Autodesk Inventor part; units mm, degrees
(part 3 of 3)
  circle A63 centre (27.5, -71.0469) radius 1.6 construction
  circle A64 centre (72.5, 11.9531) radius 1.6 construction
  circle A65 centre (27.5, 11.9531) radius 1.6 construction
  circle A66 centre (50, 69.0653) radius 1.6 construction
  arc A67 (58, 66.0653) -> (55, 66.0653) centre (56.5, 66.0653) ccw construction
  line L1375 (58, 66.0653) -> (58, 63.0653) construction
  arc A68 (55, 63.0653) -> (58, 63.0653) centre (56.5, 63.0653) ccw construction
  line L1376 (55, 63.0653) -> (45, 63.0653) construction
  arc A69 (42, 63.0653) -> (45, 63.0653) centre (43.5, 63.0653) ccw construction
  line L1377 (42, 63.0653) -> (42, 66.0653) construction
  arc A70 (45, 66.0653) -> (42, 66.0653) centre (43.5, 66.0653) ccw construction
  line L1378 (45, 66.0653) -> (55, 66.0653) construction
  circle A71 centre (50, 53.0653) radius 1.6 construction
  arc A72 (58, 50.0653) -> (55, 50.0653) centre (56.5, 50.0653) ccw construction
  line L1379 (58, 50.0653) -> (58, 47.0653) construction
  arc A73 (55, 47.0653) -> (58, 47.0653) centre (56.5, 47.0653) ccw construction
  line L1380 (55, 47.0653) -> (45, 47.0653) construction
  arc A74 (42, 47.0653) -> (45, 47.0653) centre (43.5, 47.0653) ccw construction
  line L1381 (42, 47.0653) -> (42, 50.0653) construction
  arc A75 (45, 50.0653) -> (42, 50.0653) centre (43.5, 50.0653) ccw construction
  line L1382 (45, 50.0653) -> (55, 50.0653) construction
  circle A76 centre (50, 24.7653) radius 5 construction
  circle A77 centre (50, -37.0469) radius 9.5 construction
  circle A78 centre (10, 22.9531) radius 1.6 construction
  circle A79 centre (10, -97.0469) radius 1.6 construction
  circle A80 centre (10, -97.0469) radius 1.6
  circle A81 centre (10, 47.9531) radius 1.6
  circle A82 centre (10, 22.9531) radius 1.6
  circle A83 centre (10, -122.0469) radius 1.6
  line L1383 (0, 57.9531) -> (117.0753, 93.7594)
  arc A84 (125, 92.8569) -> (125, 92.8569) centre (50, -37.0469) ccw
  arc A85 (117.0753, 93.7594) -> (125, 92.8569) centre (120, 84.1967) ccw
  circle A86 centre (50, 24.7653) radius 4
  circle A87 centre (72.5, 11.9531) radius 4
  circle A88 centre (27.5, -71.0469) radius 4
  circle A89 centre (27.5, 11.9531) radius 4
  circle A90 centre (50, -37.0469) radius 4
  line L1384 (41.6494, -157.691) -> (24.8878, -97.5563)
  line L1385 (15.5661, 31.3421) -> (117.1454, 62.4091)
  line L1386 (10, 22.9531) -> (153.2744, -98.1566) construction
  arc A91 (0, 22.9531) -> (2, 16.9531) centre (10, 22.9531) ccw
  arc A92 (146.8188, -105.7937) -> (148.6361, -107.0159) centre (153.2744, -98.1566) ccw
  line L1387 (153.2744, -98.1566) -> (10, -97.0469) construction
  arc A93 (2, -91.0469) -> (2, 16.9531) centre (-69.9999, -37.0469) ccw
  arc A94 (18, -103.0469) -> (18, 28.9531) centre (-69.9999, -37.0469) ccw
  line L1388 (117.0753, 93.7594) -> (0, 57.9531)
  line L1389 (10, -97.0469) -> (153.2744, 24.0628) construction
  arc A95 (2, -91.0469) -> (16.4556, -104.684) centre (10, -97.0469) ccw
  line L1390 (16.4556, -104.684) -> (20, -101.6879)
  arc A96 (159.73, 16.4258) -> (162.8066, 27.0857) centre (153.2744, 24.0628) ccw
  arc A97 (147.8278, 32.4494) -> (146.8188, 31.6999) centre (153.2744, 24.0628) ccw
  arc A98 (147.8278, 32.4494) -> (117.1454, 62.4091) centre (50, -37.0469) ccw
  arc A99 (154.0392, 22.7515) -> (153.2744, 24.0628) centre (50, -37.0469) ccw
  arc A100 (41.6494, -157.691) -> (148.6361, -107.0159) centre (50, -37.0469) ccw
  arc A101 (158.1017, -89.1432) -> (158.1017, 15.0494) centre (50, -37.0469) ccw
  line L1391 (24.8878, -97.5563) -> (80.9808, -50.1409)
  line L1392 (96.1463, -37.3215) -> (158.1017, 15.0494)
  line L1393 (158.1017, -89.1432) -> (96.4712, -37.0469)
  line L1394 (88.726, -30.4999) -> (85.5678, -27.8303)
  line L1395 (80.9808, -23.9529) -> (15.5661, 31.3421)
  line L1396 (146.8188, 31.6999) -> (80.9808, -23.9529)
  line L1397 (78.0566, -26.4247) -> (3.5444, -89.4098)
  line L1398 (3.5444, 15.316) -> (78.0566, -47.6691)
  line L1399 (80.9808, -50.1409) -> (146.8188, -105.7937)
  arc A102 (10.0775, -87.0472) -> (3.5444, -89.4098) centre (10, -97.0469) ccw
  arc A103 (2, -91.0469) -> (0, -97.0469) centre (10, -97.0469) ccw
  arc A104 (22.2574, -48.4638) -> (56.5973, -66.3125) centre (50, -37.0469) ccw
  arc A105 (76.5306, -51.0514) -> (72.7156, -17.451) centre (50, -37.0469) ccw
  arc A106 (69.9978, -14.6842) -> (69.3669, -14.1357) centre (50, -37.0469) ccw
  arc A107 (52.0288, -7.1156) -> (24.5, -21.2434) centre (50, -37.0469) ccw
  line L1400 (0, 57.9531) -> (0, 22.9531)
  line L1401 (0, 18.9531) -> (0, -93.0469)
  line L1402 (0, -97.0469) -> (0, -120)
  line L1403 (0, 22.9531) -> (0, -97.0469)
  point P0 (0, 0)
  point P1 (81.6372, -37.6018)
  point P2 (81.6372, -97.6018)
  point P3 (81.6372, -36.492)
extrude "押し出し7" cut sketch "スケッチ7" against normal through all contours L1384 L1391 L1399 A92 A100 | L1385 A98 A97 L1396 L1395 | A91 A93 A95 L1403 L1401 | L1393 L1392 A101
fillet "フィレット1" radius 20 11 edges at (5, -157.691, 41.6494) (5, -107.0159, 148.6361) (5, -97.5563, 24.8878) (5, -50.1409, 80.9808) (5, -37.0469, 96.4712) (5, 15.0494, 158.1017) (5, -89.1432, 158.1017) (5, -23.9529, 80.9808) (5, 31.3421, 15.5661) (5, 62.4091, 117.1454) (5, 32.4494, 147.8278)
sketch "スケッチ8" plane through (0, 0, 0) normal (-1, 0, 0) x (0, 0, 1)
  circle A0 centre (10, -160.7401) radius 1.6
  circle A1 centre (8, -136) radius 1.6
  line L0 (0, -97.0469) -> (0, -156.2222) projected
  point P0 (0, 0)
  point P1 (50, -37.0469)
  dimension "d59" = 130
  dimension "d60" = 3.2
  dimension "d61" = 10
  dimension "d62" = 3.2
  dimension "d63" = 8
  dimension "d64" = 136
  constraints: 2 centre point
  measures "d59" distance of point (50, -37.047) A0.centre
  measures "d60" diameter of A1
  measures "d61" distance from line of L0 A0.centre
  measures "d62" diameter of A0
  measures "d63" distance from line of A1.centre L0
  measures "d64" vertical distance of point (0, 0) A1.centre
extrude "押し出し8" cut sketch "スケッチ8" against normal blind 10
fillet "フィレット2" radius 20 1 edges at (5, 57.9531, 0)
sketch "スケッチ9" plane through (0, 0, 0) normal (-1, 0, 0) x (0, 0, 1)
  line L0 (8, -85.5469) -> (1, -85.5469) projected
  line L1 (1, -85.5469) -> (1, -78.5469) projected
  line L2 (1, -78.5469) -> (8, -78.5469) projected
  line L3 (8, -78.5469) -> (8, -85.5469) projected
  line L4 (9, -86.5469) -> (9, -77.5469) projected
  line L5 (9, -77.5469) -> (0, -77.5469) projected
  line L6 (0, -77.5469) -> (0, -86.5469) projected
  line L7 (0, -86.5469) -> (9, -86.5469) projected
  line L8 (184, -74.5469) -> (178, -74.5469)
  line L9 (175, -74.5469) -> (175, -77.5469)
  line L10 (178, -77.5469) -> (184, -77.5469)
  line L11 (187, -77.5469) -> (187, -74.5469)
  arc A0 (178, -74.5469) -> (175, -74.5469) centre (176.5, -74.5469) ccw
  arc A1 (175, -77.5469) -> (178, -77.5469) centre (176.5, -77.5469) ccw
  arc A2 (184, -77.5469) -> (187, -77.5469) centre (185.5, -77.5469) ccw
  arc A3 (187, -74.5469) -> (184, -74.5469) centre (185.5, -74.5469) ccw
  line L12 (8, 4.4531) -> (1, 4.4531) projected
  line L13 (1, 4.4531) -> (1, 11.4531) projected
  line L14 (1, 11.4531) -> (8, 11.4531) projected
  line L15 (8, 11.4531) -> (8, 4.4531) projected
  line L16 (9, 3.4531) -> (9, 12.4531) projected
  line L17 (9, 12.4531) -> (0, 12.4531) projected
  line L18 (0, 12.4531) -> (0, 3.4531) projected
  line L19 (0, 3.4531) -> (9, 3.4531) projected
  line L20 (184, 3.4531) -> (178, 3.4531)
  line L21 (175, 3.4531) -> (175, 0.4531)
  arc A4 (178, 3.4531) -> (175, 3.4531) centre (176.5, 3.4531) ccw
  arc A5 (175, 0.4531) -> (178, 0.4531) centre (176.5, 0.4531) ccw
  arc A6 (187, 3.4531) -> (184, 3.4531) centre (185.5, 3.4531) ccw
  line L22 (187, 0.4531) -> (187, 3.4531)
  arc A7 (184, 0.4531) -> (187, 0.4531) centre (185.5, 0.4531) ccw
  line L23 (178, 0.4531) -> (184, 0.4531)
  point P0 (0, 0)
  dimension "d41" = 3
  dimension "d42" = 12
  dimension "d43" = 166
  dimension "d44" = 3
  dimension "d45" = 3
  dimension "d46" = 3
  dimension "d47" = 3
  dimension "d52" = 78
  constraints: 16 end point, 16 point on circle, 16 point on line, 8 centre point, 2 collinear, 2 parallel, 1 horizontal, 1 perpendicular, 1 vertical, 19 other
  measures "d41" distance of L11.start L11.end
  measures "d42" distance of L9.end L11.start
  measures "d43" distance between parallel lines of L4 L9
  measures "d44" diameter of A0
  measures "d45" diameter of A1
  measures "d46" diameter of A2
  measures "d47" diameter of A3
  measures "d52" distance of L11.end L22.end
extrude "押し出し9" cut sketch "スケッチ9" against normal through all contours A3 L11 A2 L10 A1 L9 A0 L8 | A6 L22 A7 L23 A5 L21 A4 L20
sketch "スケッチ10" plane through (0, 0, 0) normal (-1, 0, 0) x (0, 0, 1)
  circle A0 centre (160.3684, -95.7308) radius 1.6 projected
  circle A1 centre (165.898, -83.8727) radius 1.6 projected
  circle A2 centre (8, -136) radius 1.6 projected
  arc A3 (40, -166.6617) -> (159.9522, -106.4048) centre (50, -37.0469) ccw projected
  arc A4 (159.9522, -106.4048) -> (158.3435, -101.9515) centre (157.4148, -104.8042) ccw projected
  arc A5 (163.1332, -89.8018) -> (158.3435, -101.9515) centre (160.3684, -95.7308) ccw projected
  arc A6 (169.3617, -78.3229) -> (163.1332, -89.8018) centre (165.898, -83.8727) ccw projected
  arc A7 (169.3617, -78.3229) -> (173.8071, -76.6928) centre (170.95, -75.7779) ccw projected
  arc A8 (173.8071, -76.6928) -> (165.0418, 23.4956) centre (50, -37.0469) ccw projected
  arc A9 (165.0418, 23.4956) -> (160.3808, 24.329) centre (162.387, 22.0984) ccw projected
  arc A10 (152.2537, 34.5519) -> (160.3808, 24.329) centre (156.006, 29.193) ccw projected
  arc A11 (145.4269, 45.6854) -> (152.2537, 34.5519) centre (148.5013, 39.9108) ccw projected
  arc A12 (145.4269, 45.6854) -> (146.2379, 50.3503) centre (144.017, 48.3334) ccw projected
  arc A13 (146.2379, 50.3503) -> (115, 75.5364) centre (50, -37.0469) ccw projected
  arc A14 (125, 92.8569) -> (115, 75.5364) centre (120, 84.1967) ccw projected
  arc A15 (23.9528, -184.768) -> (125, 92.8569) centre (50, -37.0469) ccw projected
  arc A16 (15.7254, -174.0707) -> (23.9528, -184.768) centre (25.6893, -174.92) ccw projected
  arc A17 (15.7254, -174.0707) -> (4.8819, -138.5055) centre (-34.094, -169.8245) ccw projected
  arc A18 (9.8395, -132.448) -> (4.8819, -138.5055) centre (8, -136) ccw projected
  arc A19 (34.717, -162.4118) -> (9.8395, -132.448) centre (-13.1537, -176.8475) ccw projected
  arc A20 (34.717, -162.4118) -> (40, -166.6617) centre (40.4615, -160.6795) ccw projected
  circle A21 centre (148.5013, 39.9108) radius 1.6 projected
  circle A22 centre (156.006, 29.193) radius 1.6 projected
  circle A23 centre (120, 84.1967) radius 1.6 projected
extrude "押し出し10" cut sketch "スケッチ10" against normal blind 10 contours A0 | A1 | A21 | A22
sketch "スケッチ11" plane through (0, 0, 0) normal (-1, 0, 0) x (0, 0, 1)
  arc A0 (187, -74.5469) -> (184, -74.5469) centre (185.5, -74.5469) ccw projected
  line L0 (187, -74.5469) -> (187, -77.5469) projected
  arc A1 (184, -77.5469) -> (187, -77.5469) centre (185.5, -77.5469) ccw projected
  line L1 (184, -77.5469) -> (178, -77.5469) projected
  arc A2 (175, -77.5469) -> (178, -77.5469) centre (176.5, -77.5469) ccw projected
  line L2 (175, -77.5469) -> (175, -74.5469) projected
  arc A3 (178, -74.5469) -> (175, -74.5469) centre (176.5, -74.5469) ccw projected
  line L3 (178, -74.5469) -> (184, -74.5469) projected
  arc A4 (187, 3.4531) -> (184, 3.4531) centre (185.5, 3.4531) ccw projected
  line L4 (187, 3.4531) -> (187, 0.4531) projected
  arc A5 (184, 0.4531) -> (187, 0.4531) centre (185.5, 0.4531) ccw projected
  line L5 (184, 0.4531) -> (178, 0.4531) projected
  arc A6 (175, 0.4531) -> (178, 0.4531) centre (176.5, 0.4531) ccw projected
  line L6 (175, 0.4531) -> (175, 3.4531) projected
  arc A7 (178, 3.4531) -> (175, 3.4531) centre (176.5, 3.4531) ccw projected
  line L7 (178, 3.4531) -> (184, 3.4531) projected
  line L8 (68.0695, -13.039) -> (43.573, 7.6679) projected
  arc A8 (50.6349, 42.0676) -> (43.573, 7.6679) centre (56.4842, 22.9421) ccw projected
  line L9 (50.6349, 42.0676) -> (107.4949, 59.4576) projected
  arc A9 (126.0131, 55.8079) -> (107.4949, 59.4576) centre (113.3442, 40.3321) ccw projected
  arc A10 (133.4389, 49.1967) -> (126.0131, 55.8079) centre (50, -37.0469) ccw projected
  arc A11 (132.4436, 19.5486) -> (133.4389, 49.1967) centre (119.5324, 34.8228) ccw projected
  line L10 (132.4436, 19.5486) -> (93.892, -13.039) projected
  arc A12 (68.0695, -13.039) -> (93.892, -13.039) centre (80.9808, 2.2351) ccw projected
  line L11 (114.5407, -21.7727) -> (135.5059, -4.0509) projected
  arc A13 (168.1006, -15.7806) -> (135.5059, -4.0509) centre (148.4172, -19.325) ccw projected
  arc A14 (168.1006, -58.3132) -> (168.1006, -15.7806) centre (50, -37.0469) ccw projected
  arc A15 (135.5059, -70.0429) -> (168.1006, -58.3132) centre (148.4171, -54.7688) ccw projected
  line L12 (135.5059, -70.0429) -> (114.5407, -52.3211) projected
  arc A16 (114.5407, -21.7727) -> (114.5407, -52.3211) centre (127.4519, -37.0469) ccw projected
  arc A17 (58.2105, -157.7006) -> (134.1681, -123.8827) centre (50, -37.0469) ccw projected
  arc A18 (37.587, -143.1167) -> (58.2105, -157.7006) centre (56.8526, -137.7468) ccw projected
  line L13 (37.587, -143.1167) -> (28.3331, -109.9168) projected
  arc A19 (34.6874, -89.2726) -> (28.3331, -109.9168) centre (47.5987, -104.5468) ccw projected
  line L14 (34.6874, -89.2726) -> (68.0695, -61.0548) projected
  arc A20 (93.892, -61.0548) -> (68.0695, -61.0548) centre (80.9808, -76.3289) ccw projected
  line L15 (93.892, -61.0548) -> (133.1595, -94.2476) projected
  arc A21 (134.1681, -123.8827) -> (133.1595, -94.2476) centre (120.2483, -109.5217) ccw projected
  circle A22 centre (10, -97.0469) radius 1.6 projected
  circle A23 centre (10, 47.9531) radius 1.6 projected
  circle A24 centre (10, 22.9531) radius 1.6 projected
  circle A25 centre (10, -122.0469) radius 1.6 projected
  arc A26 (14.1507, 62.281) -> (0, 43.1554) centre (20, 43.1554) ccw projected
  line L16 (0, 43.1554) -> (0, 22.9531) projected
  arc A27 (0, 22.9531) -> (2, 16.9531) centre (10, 22.9531) ccw projected
  arc A28 (2, -91.0469) -> (2, 16.9531) centre (-69.9999, -37.0469) ccw projected
  arc A29 (2, -91.0469) -> (0, -97.0469) centre (10, -97.0469) ccw projected
  line L17 (0, -97.0469) -> (0, -156.2222) projected
  arc A30 (0, -156.2222) -> (23.9528, -184.768) centre (28.9862, -156.2222) ccw projected
  arc A31 (23.9528, -184.768) -> (125, 92.8569) centre (50, -37.0469) ccw projected
  arc A32 (125, 92.8569) -> (117.0753, 93.7594) centre (120, 84.1967) ccw projected
  line L18 (14.1507, 62.281) -> (117.0753, 93.7594) projected
  circle A33 centre (27.5, -71.0469) radius 4 projected
  circle A34 centre (27.5, 11.9531) radius 4 projected
  circle A35 centre (50, -37.0469) radius 4 projected
  circle A36 centre (8, -136) radius 1.6 projected
  circle A37 centre (10, -160.7401) radius 1.6 projected
  arc A38 (0, -128.2058) -> (2.6711, -133.1976) centre (6, -128.2058) ccw
  line L19 (0, -97.0469) -> (0, -156.2222) projected
  arc A39 (0, -156.2222) -> (23.9528, -184.768) centre (28.9862, -156.2222) ccw projected
  circle A40 centre (8, -136) radius 4
  circle A41 centre (160.3684, -95.7308) radius 1.6 projected
  circle A42 centre (165.898, -83.8727) radius 1.6 projected
  circle A43 centre (8, -136) radius 1.6 projected
  arc A44 (40, -166.6617) -> (159.9522, -106.4048) centre (50, -37.0469) ccw projected
  arc A45 (159.9522, -106.4048) -> (158.3435, -101.9515) centre (157.4148, -104.8042) ccw projected
  arc A46 (163.1332, -89.8018) -> (158.3435, -101.9515) centre (160.3684, -95.7308) ccw projected
  arc A47 (169.3617, -78.3229) -> (163.1332, -89.8018) centre (165.898, -83.8727) ccw projected
  arc A48 (169.3617, -78.3229) -> (173.8071, -76.6928) centre (170.95, -75.7779) ccw projected
  arc A49 (173.8071, -76.6928) -> (165.0418, 23.4956) centre (50, -37.0469) ccw projected
  arc A50 (165.0418, 23.4956) -> (160.3808, 24.329) centre (162.387, 22.0984) ccw projected
  arc A51 (152.2537, 34.5519) -> (160.3808, 24.329) centre (156.006, 29.193) ccw projected
  arc A52 (145.4269, 45.6854) -> (152.2537, 34.5519) centre (148.5013, 39.9108) ccw projected
  arc A53 (145.4269, 45.6854) -> (146.2379, 50.3503) centre (144.017, 48.3334) ccw projected
  arc A54 (146.2379, 50.3503) -> (115, 75.5364) centre (50, -37.0469) ccw projected
  arc A55 (125, 92.8569) -> (115, 75.5364) centre (120, 84.1967) ccw projected
  arc A56 (23.9528, -184.768) -> (125, 92.8569) centre (50, -37.0469) ccw projected
  arc A57 (15.7254, -174.0707) -> (23.9528, -184.768) centre (25.6893, -174.92) ccw projected
  arc A58 (15.7254, -174.0707) -> (4.8819, -138.5055) centre (-34.094, -169.8245) ccw projected
  arc A59 (9.8395, -132.448) -> (4.8819, -138.5055) centre (8, -136) ccw projected
  arc A60 (34.717, -162.4118) -> (9.8395, -132.448) centre (-13.1537, -176.8475) ccw projected
  arc A61 (34.717, -162.4118) -> (40, -166.6617) centre (40.4615, -160.6795) ccw projected
  circle A62 centre (148.5013, 39.9108) radius 1.6 projected
  circle A63 centre (156.006, 29.193) radius 1.6 projected
  arc A64 (4.0038, -135.8249) -> (2.6711, -133.1976) centre (1.0067, -135.6936) ccw
  circle A65 centre (120, 84.1967) radius 1.6 projected
  point P0 (0, 0)
  dimension "d67" = 6
  dimension "d74" = 8
  dimension "d75" = 3
  constraints: 5 point on circle, 3 centre point, 3 tangent, 1 coincident, 1 point on line
  measures "d67" radius of A38
  measures "d74" diameter of A40
  measures "d75" radius of A64
extrude "押し出し11" cut sketch "スケッチ11" against normal blind 10 contours A30 L17 A38 A64 A40 A58 A57 | A37
